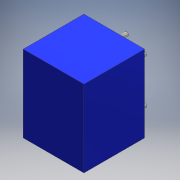
# Autodesk Inventor part: miniRelay
Saved by Autodesk Inventor 2016 (Build 200138000, 138)
## iProperties
Created: 2015-11-01
Part Number: miniRelay
Material: Generic
Document SubType Name: Modeling
Designer: Artur
Density: 1 g/cm^3
Appearance: Default
Mass: 4.28678 g
Surface Area: 16.3712 cm^2
Volume: 4.28678 cm^3
Author: Artur
Autodesk Inventor part; units mm, degrees
ref_plane "YZ Plane" through (0, 0, 0) normal (1, 0, 0) x (0, 1, 0)
ref_plane "XZ Plane" through (0, 0, 0) normal (0, 1, 0) x (-1, 0, 0)
ref_plane "XY Plane" through (0, 0, 0) normal (0, 0, 1) x (1, 0, 0)
sketch "Sketch1" plane through (0, 0, 0) normal (0, 1, 0) x (-1, 0, 0)
  line L0 (0, 0) -> (15, 0)
  line L1 (15, 0) -> (15, -19)
  line L2 (15, -19) -> (0, -19)
  line L3 (0, -19) -> (0, 0)
  dimension "d0" = 19
  dimension "d1" = 15
  constraints: 8 end point, 2 parallel, 1 horizontal, 1 perpendicular
  measures "d0" distance of L0.end L1.end
  measures "d1" distance of L1.end L2.end
extrude "Extrusion1" add sketch "Sketch1" along normal blind 15
sketch "Sketch2" plane through (0, 15, 0) normal (0, 1, 0) x (1, 0, 0)
  circle A0 centre (-3, 4) radius 0.5
  line L0 (0, 0) -> (0, 19) projected
  line L1 (-15, 0) -> (0, 0) projected
  circle A1 centre (-3, 15) radius 0.5
  line L2 (0, 19) -> (-15, 19) projected
  circle A2 centre (-7.5, 2) radius 0.5
  line L3 (-7.5, 0) -> (-7.5, 19) construction
  circle A3 centre (-12, 4) radius 0.5
  circle A4 centre (-12, 15) radius 0.5
  dimension "d4" = 1
  dimension "d5" = 3
  dimension "d6" = 4
  dimension "d7" = 1
  dimension "d8" = 3
  dimension "d9" = 4
  dimension "d10" = 1
  dimension "d11" = 2
  constraints: 5 centre point, 2 end point, 2 midpoint, 2 symmetric about line, 1 point on line, 2 other
  measures "d4" diameter of A0
  measures "d5" distance from line of L0 A0.centre
  measures "d6" distance from line of L1 A0.centre
  measures "d7" diameter of A1
  measures "d8" distance from line of L0 A1.centre
  measures "d9" distance from line of L2 A1.centre
  measures "d10" diameter of A2
  measures "d11" distance from line of L1 A2.centre
extrude "Extrusion2" add sketch "Sketch2" along normal blind 3
sketch "Sketch3" plane through (-12, 18, -4) normal (0, 1, 0) x (1, 0, 0)
  circle A0 centre (4.5, -2) radius 0.5 projected
  circle A1 centre (9, 0) radius 0.5 projected
  circle A2 centre (9, 11) radius 0.5 projected
  circle A3 centre (0, 0) radius 0.5 projected
  circle A4 centre (0, 11) radius 0.5 projected
  point P0 (12, -4)
  constraints: 5 coincident
body "Solid1"
